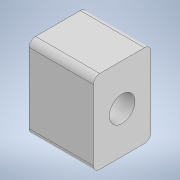
# Autodesk Inventor part: Soporte placa B1 - B2
Saved by Autodesk Inventor 2020 (Build 240168000, 168)
## iProperties
Created: 2020-05-18
Part Number: Soporte placa B1 - B2
Material: Genérico
Document SubType Name: Modeling
Designer: javic
Density: 1 g/cm^3
Appearance: Valor por defecto
Author: javic
Autodesk Inventor part; units mm, degrees
ref_plane "YZ Plane" through (0, 0, 0) normal (1, 0, 0) x (0, 1, 0)
ref_plane "XZ Plane" through (0, 0, 0) normal (0, 1, 0) x (-1, 0, 0)
ref_plane "XY Plane" through (0, 0, 0) normal (0, 0, 1) x (1, 0, 0)
sketch "Boceto3" plane through (0, 0, 0) normal (1, 0, 0) x (0, 1, 0)
  line L0 (0, 0) -> (0, -9)
  line L1 (0, -9) -> (13, -9)
  line L2 (13, -9) -> (13, 0)
  line L3 (13, 0) -> (0, 0)
  circle A0 centre (6.5, -4.5) radius 0.9
  dimension "d3" = 9
  dimension "d4" = 13
  dimension "d7" = 1.8
  constraints: 8 end point, 3 perpendicular, 1 centre point, 1 vertical
  measures "d3" distance of L0.start L0.end
  measures "d4" distance of L0.end L1.end
  measures "d7" diameter of A0
extrude "Extrusión1" add sketch "Boceto3" along normal blind 10.06
sketch "Boceto4" plane through (10.06, 0, 0) normal (1, 0, 0) x (0, 0, -1)
  point P0 (0, 0)
  point P1 (4.4995, 6.4877)
hole "Agujero1" at (10.06, 6.4877, -4.4995) direction (-1, 0, 0) diameter 4 depth 9
fillet "Empalme1" radius 1 4 edges at (5.03, 13, 0) (5.03, 13, -9) (5.03, 0, 0) (5.03, 0, -9)
